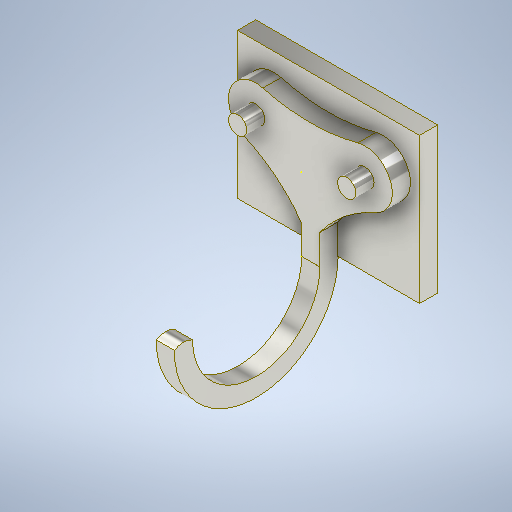
# Autodesk Inventor part: cad@25
Saved by Autodesk Inventor 2025.2 (Build 292293000, 293)
## iProperties
Created: 2025-03-15
Part Number: cad@25
Material: Generic
Document SubType Name: Modeling
Designer: spars
Density: 1 g/cm^3
Appearance: Silver
Author: spars
Autodesk Inventor part; units mm, degrees
ref_plane "YZ Plane" through (0, 0, 0) normal (1, 0, 0) x (0, 1, 0)
ref_plane "XZ Plane" through (0, 0, 0) normal (0, 1, 0) x (-1, 0, 0)
ref_plane "XY Plane" through (0, 0, 0) normal (0, 0, 1) x (1, 0, 0)
sketch "Sketch1" plane through (0, 0, 0) normal (0, 0, 1) x (1, 0, 0)
  line L0 (-10, 8) -> (10, 8)
  line L1 (10, 8) -> (10, -8)
  line L2 (10, -8) -> (-10, -8)
  line L3 (-10, -8) -> (-10, 8)
  line L4 (-10, 8) -> (10, -8) construction
  line L5 (10, 8) -> (-10, -8) construction
  point P0 (0, 0)
  dimension "d0" = 20
  dimension "d1" = 16
  constraints: 12 end point, 2 midpoint, 2 parallel, 1 horizontal, 1 perpendicular
  measures "d0" distance of L1.end L2.end
  measures "d1" distance of L0.end L1.end
extrude "Extrusion1" add sketch "Sketch1" along normal blind 2
sketch "Sketch2" plane through (0, 0, 2) normal (0, 0, 1) x (1, 0, 0)
  line L0 (10, 8) -> (-10, 8) projected
  line L1 (0, -0.2535) -> (0, 8)
  line L2 (0, 0) -> (0, -7.9613)
  line L3 (-10, -8) -> (10, -8) projected
  arc A0 (-5.2174, 5.8961) -> (-7.1982, 0.2497) centre (-6, 3) ccw
  arc A1 (7.1982, 0.2497) -> (5.2174, 5.8961) centre (6, 3) ccw
  arc A2 (-5.2174, 5.8961) -> (5.2174, 5.8961) centre (0, 25.2036) ccw
  line L4 (21.5208, 4.9837) -> (21.5208, 0.7791)
  line L5 (-1, -4.7601) -> (-1, -8)
  line L6 (1, -4.7601) -> (1, -8)
  arc A3 (-1, -4.7601) -> (-7.1982, 0.2497) centre (-13.1894, -13.5019) ccw
  arc A4 (7.1982, 0.2497) -> (1, -4.7601) centre (13.1894, -13.5019) ccw
  dimension "d8" = 16
  dimension "d14" = 15.5208
  dimension "d15" = 27.5208
  dimension "d16" = 1
  dimension "d18" = 15
  constraints: 10 end point, 10 point on circle, 5 centre point, 4 symmetric about line, 3 point on line, 3 tangent, 2 vertical, 1 midpoint, 1 perpendicular, 2 other
  measures "d8" distance between parallel lines of L3 L0
  measures "d14" distance from line of L4 A1.centre
  measures "d15" distance from line of L4 A0.centre
  measures "d16" distance between parallel lines of L5 L2
  measures "d18" radius of A3
extrude "Extrusion2" add sketch "Sketch2" along normal blind 2
sketch "Sketch3" plane through (0, 0, 4) normal (0, 0, 1) x (1, 0, 0)
  circle A0 centre (-6, 3) radius 1
  line L0 (10, 8) -> (-10, 8) projected
  circle A1 centre (6, 3) radius 1
  point P0 (0, 0)
  dimension "d21" = 2
  dimension "d22" = 5
  constraints: 2 centre point
  measures "d21" diameter of A0
  measures "d22" distance from line of L0 A0.centre
extrude "Extrusion3" add sketch "Sketch3" along normal blind 2
sketch "Sketch4" plane through (0, 0, 0) normal (0, 1, 0) x (-1, 0, 0)
  point P0 (0, 0)
sketch "Sketch5" plane through (0, 0, 0) normal (1, 0, 0) x (0, 1, 0)
  point P0 (0, 0)
sketch "Sketch6" plane through (-10, -8, 0) normal (0, -1, 0) x (1, 0, 0)
  line L0 (9, 2) -> (9, 4) projected
  point P0 (10, 0)
sketch "Sketch7" plane through (-10, -8, 0) normal (0, -1, 0) x (1, 0, 0)
  point P0 (10, 0)
sketch "Sketch8" plane through (0, 0, 0) normal (1, 0, 0) x (0, 1, 0)
  point P0 (0, 0)
sketch "Sketch9" plane through (0, 0, 0) normal (0, 0, 1) x (1, 0, 0)
  point P0 (0, 0)
extrude "Extrusion4" [suppressed]
sketch "Sketch10" plane through (0, 0, 0) normal (0, 1, 0) x (-1, 0, 0)
  point P0 (0, 0)
sketch "Sketch11" plane through (0, 0, 0) normal (0, 1, 0) x (-1, 0, 0)
  point P0 (0, 0)
extrude "Extrusion5" [suppressed]
sketch "Sketch12" plane through (0, 0, 0) normal (1, 0, 0) x (0, 1, 0)
  point P0 (0, 0)
sketch "Sketch13" plane through (0, 0, 0) normal (0, 1, 0) x (-1, 0, 0)
  line L0 (1, 2) -> (1, 4) projected
  point P0 (0, 0)
sketch "Sketch14" plane through (0, 0, 0) normal (0, 1, 0) x (-1, 0, 0)
  point P0 (0, 0)
extrude "Extrusion6" [suppressed]
sketch "Sketch15" plane through (0, 0, 0) normal (1, 0, 0) x (0, 1, 0)
  arc A0 (-7.985, 19.9445) -> (-7.985, 1.9445) centre (-7.985, 10.9445) ccw
  arc A1 (-7.985, 17.9445) -> (-7.985, 3.9445) centre (-7.985, 10.9445) ccw
  line L0 (-7.985, 1.9445) -> (-7.985, 3.9445)
  arc A2 (-7.985, 17.9445) -> (-7.985, 19.9445) centre (-9.717, 18.9445) ccw
  point P0 (0, 0)
  dimension "d44" = 2
  constraints: 6 point on circle, 3 centre point, 2 end point, 1 coincident, 1 vertical
  measures "d44" radius of A2
extrude "Extrusion7" add sketch "Sketch15" along normal mid plane 2
body "Solid1"
